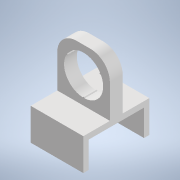
# Autodesk Inventor part: Sujetador_Carril
Saved by Autodesk Inventor 2022 (Build 260153000, 153)
## iProperties
Created: 2022-01-30
Part Number: Sujetador_Carril
Material: Generic
Document SubType Name: Modeling
Designer: katha
Density: 1 g/cm^3
Appearance: Default
Author: katha
Autodesk Inventor part; units mm, degrees
ref_plane "YZ Plane" through (0, 0, 0) normal (1, 0, 0) x (0, 1, 0)
ref_plane "XZ Plane" through (0, 0, 0) normal (0, 1, 0) x (-1, 0, 0)
ref_plane "XY Plane" through (0, 0, 0) normal (0, 0, 1) x (1, 0, 0)
sketch "Sketch2" plane through (0, 0, 0) normal (1, 0, 0) x (0, 1, 0)
  line L0 (0, -12.532) -> (0, 12.468) projected
  line L1 (0, 12.468) -> (3, 12.468) projected
  line L2 (3, -12.532) -> (3, 12.468) projected
  line L3 (0, -12.532) -> (3, -12.532) projected
  line L4 (-17, -12.532) -> (3, -12.532) projected
  line L5 (3, -12.532) -> (3, -15.532) projected
  line L6 (-17, -15.532) -> (3, -15.532) projected
  line L7 (-17, -12.532) -> (-17, -15.532) projected
  line L8 (3.3, -13.032) -> (3.3, -0.032)
  line L9 (-14.7, -15.832) -> (3.3, -15.832)
  line L10 (3.3, -13.032) -> (3.3, -15.832)
  line L11 (-14.7, -18.832) -> (6.5, -18.832)
  line L12 (3.3, -0.032) -> (6.5, -0.032) construction
  line L13 (-14.7, -15.832) -> (-14.7, -18.832)
  line L14 (36.5, -3.682) -> (6.5, -3.682)
  line L15 (3.3, 12.968) -> (3.3, -0.032)
  line L16 (-14.7, 15.768) -> (3.3, 15.768)
  line L17 (3.3, 12.968) -> (3.3, 15.768)
  line L18 (-14.7, 18.768) -> (6.5, 18.768)
  line L19 (-14.7, 15.768) -> (-14.7, 18.768)
  line L20 (36.5, 3.618) -> (6.5, 3.618)
  line L21 (3, 12.468) -> (-17, 12.468) projected
  line L22 (-17, 12.468) -> (-17, 15.468) projected
  line L23 (3, 15.468) -> (-17, 15.468) projected
  line L24 (3, 12.468) -> (3, 15.468) projected
  line L25 (6.5, 18.768) -> (6.5, 3.618)
  line L26 (6.5, -18.832) -> (6.5, -3.682)
  line L27 (36.5, 3.618) -> (36.5, -3.682)
  point P0 (0, 0)
  dimension "d0" = 0.3
  dimension "d1" = 0.3
  dimension "d3" = 18
  dimension "d4" = 3
  dimension "d11" = 3.5
  dimension "d33" = 7.3
  dimension "d34" = 30
  dimension "d35" = 15.15
  constraints: 32 end point, 7 symmetric about line, 3 vertical, 2 perpendicular
  measures "d0" distance between parallel lines of L2 L8
  measures "d1" distance between parallel lines of L6 L9
  measures "d3" distance between parallel lines of L13 L10
  measures "d4" distance between parallel lines of L11 L9
  measures "d11" distance between parallel lines of L26 L2
  measures "d33" distance between parallel lines of L14 L20
  measures "d34" distance of L14.start L14.end
  measures "d35" distance between parallel lines of L11 L14
extrude "Extrusion1" add sketch "Sketch2" along normal blind 15 and the other way blind 15 contours L8 L15 L17 L16 L19 L18 L25 L20 L27 L14 L26 L11 L13 L9 L10
sketch "Sketch5" plane through (15, 36.5, -3.682) normal (0, 0, -1) x (-1, 0, 0)
  line L0 (30, -30) -> (0, -30) projected
  line L1 (30, 0) -> (0, 0) projected
  line L2 (0, -30) -> (30, -30) projected
  line L3 (30, 0) -> (0, 0) projected
  arc A0 (15.4999, -26.1388) -> (14.5001, -26.1388) centre (15, -26.15) ccw
  arc A1 (24.3965, -8.9977) -> (24.8964, -9.8635) centre (24.6562, -9.425) ccw
  arc A2 (5.1036, -9.8635) -> (5.6035, -8.9977) centre (5.3438, -9.425) ccw
  arc A3 (15.4999, -26.1388) -> (24.8964, -9.8635) centre (15, -15) ccw
  arc A4 (24.3965, -8.9977) -> (5.6035, -8.9977) centre (15, -15) ccw
  arc A5 (5.1036, -9.8635) -> (14.5001, -26.1388) centre (15, -15) ccw
  point P0 (15, -36.5)
  dimension "d37" = 1
  dimension "d40" = 360
  dimension "d42" = 15
  dimension "d43" = 15
  dimension "d44" = 11.15
  constraints: 12 point on circle, 6 centre point, 13 other
  measures "d37" diameter of A0
  measures "d42" distance from line of A3.centre L0
  measures "d43" horizontal distance of L1.end A3.centre
  measures "d44" radius of A3
extrude "Extrusion2" cut sketch "Sketch5" against normal blind 10
fillet "Fillet2" radius 11 2 edges at (-15, 36.5, -0.032) (15, 36.5, -0.032)
sketch "Sketch7" plane through (15, 6.5, -18.832) normal (0, 0, -1) x (-1, 0, 0)
  circle A0 centre (15, -15.7) radius 2 projected
  circle A1 centre (15, -15.7) radius 2
  point P0 (15, -6.5)
  constraints: 1 centre point, 1 coincident, 1 concentric
extrude "Extrusion4" cut sketch "Sketch7" against normal blind 40
body "Solid1"
